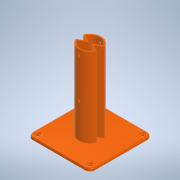
# Autodesk Inventor part: Arduino_case_top_JC_Rev1
Saved by Autodesk Inventor 2020 (Build 240168000, 168)
## iProperties
Created: 2019-08-28
Part Number: Arduino_case_top_JC_Rev1
Material: Generic
Document SubType Name: Modeling
Designer: jcocker
Density: 1 g/cm^3
Appearance: Smooth - Light Orange
Author: jcocker
Autodesk Inventor part; units mm, degrees
ref_plane "YZ Plane" through (0, 0, 0) normal (1, 0, 0) x (0, 1, 0)
ref_plane "XZ Plane" through (0, 0, 0) normal (0, 1, 0) x (-1, 0, 0)
ref_plane "XY Plane" through (0, 0, 0) normal (0, 0, 1) x (1, 0, 0)
sketch "Sketch1" plane through (0, 0, 0) normal (0, 1, 0) x (-1, 0, 0)
  circle A0 centre (0, 0) radius 14.2875
  line L0 (5.08, 0) -> (13.4462, -4.8303)
  line L1 (5.08, 0) -> (14.7405, 0) construction
  line L2 (5.08, 0) -> (13.4462, 4.8303)
  line L3 (-5.08, 0) -> (-13.4462, -4.8303)
  line L4 (-5.08, 0) -> (-13.4462, 4.8303)
  dimension "d0" = 28.575
  dimension "d1" = 5.08
  dimension "d2" = 30
  constraints: 10 end point, 1 coincident, 1 equal length, 1 horizontal, 1 symmetric about line, 3 other
  measures "d1" distance of point (0, 0) L0.start
  measures "d2" angle of L0 L1
extrude "Extrusion1" add sketch "Sketch1" along normal blind 101.6 contours L2 L0 A0 L3 L4
shell "Shell1" thickness 1.7 removed faces 2 at (0, 0, -4.7625) at (0, 101.6, -4.7625)
sketch "Sketch2" plane through (0, 0, 0) normal (0, -1, 0) x (1, 0, 0)
  line L0 (33.65, 40) -> (-33.65, 40)
  line L1 (-40, 33.65) -> (-40, -33.65)
  line L2 (-33.65, -40) -> (33.65, -40)
  line L3 (40, -33.65) -> (40, 33.65)
  line L4 (40, 40) -> (-40, -40) construction
  line L5 (-40, 40) -> (40, -40) construction
  arc A0 (33.65, -40) -> (40, -33.65) centre (33.65, -33.65) ccw
  arc A1 (40, 33.65) -> (33.65, 40) centre (33.65, 33.65) ccw
  arc A2 (-33.65, 40) -> (-40, 33.65) centre (-33.65, 33.65) ccw
  arc A3 (-40, -33.65) -> (-33.65, -40) centre (-33.65, -33.65) ccw
  point P0 (0, 0)
  dimension "d6" = 80
  dimension "d7" = 80
  dimension "d9" = 6.35
  constraints: 12 end point, 8 point on circle, 8 point on line, 8 tangent, 4 centre point, 3 equal radius, 2 midpoint, 2 parallel, 1 horizontal, 1 perpendicular
  measures "d6" distance of L5.end L4.end
  measures "d7" distance of L4.end L5.start
  measures "d9" radius of A0
extrude "Extrusion2" add sketch "Sketch2" along normal blind 3.175
sketch "Sketch3" plane through (0, 0, 0) normal (0, 1, 0) x (1, 0, 0)
  arc A0 (-11.2968, -5.5523) -> (11.2968, -5.5523) centre (0, 0) ccw projected
  line L0 (11.2968, -5.5523) -> (1.68, 0) projected
  line L1 (1.68, 0) -> (11.2968, 5.5523) projected
  arc A1 (11.2968, 5.5523) -> (-11.2968, 5.5523) centre (0, 0) ccw projected
  line L2 (-11.2968, 5.5523) -> (-1.68, 0) projected
  line L3 (-1.68, 0) -> (-11.2968, -5.5523) projected
extrude "Extrusion3" cut sketch "Sketch3" against normal through all
sketch "Sketch4" plane through (0, 0, 0) normal (0, 0, 1) x (1, 0, 0)
  circle A0 centre (0, 44.45) radius 1.5875
  point P0 (0, 0)
  dimension "d14" = 3.175
  dimension "d15" = 44.45
  constraints: 1 centre point
  measures "d14" diameter of A0
  measures "d15" distance of point (0, 0) A0.centre
extrude "Extrusion4" cut sketch "Sketch4" along normal mid plane 101.6
sketch "Sketch5" plane through (0, 0, 0) normal (0, 0, 1) x (1, 0, 0)
  circle A0 centre (0, 95.25) radius 1.5875
  line L0 (33.65, 0) -> (40, 0) projected
  point P0 (0, 0)
  dimension "d18" = 3.175
  dimension "d19" = 95.25
  constraints: 1 centre point
  measures "d18" diameter of A0
  measures "d19" distance from line of L0 A0.centre
extrude "Extrusion5" cut sketch "Sketch5" along normal blind 101.6 and the other way blind 50.8
sketch "Sketch6" plane through (0, 0, 0) normal (0, 1, 0) x (1, 0, 0)
  arc A0 (40, 33.65) -> (33.65, 40) centre (33.65, 33.65) ccw projected
  circle A1 centre (33.65, 33.65) radius 1.7
  point P0 (0, 0)
  dimension "d24" = 3.4
  constraints: 1 centre point, 1 coincident
  measures "d24" diameter of A1
extrude "Extrusion6" cut sketch "Sketch6" against normal blind 25.4
sketch "Sketch7" plane through (0, 0, 0) normal (0, 1, 0) x (1, 0, 0)
  arc A0 (40, 33.65) -> (33.65, 40) centre (33.65, 33.65) ccw projected
  circle A1 centre (33.65, 33.65) radius 3.175
  point P0 (0, 0)
  dimension "d27" = 6.35
  constraints: 1 centre point, 1 coincident
  measures "d27" diameter of A1
extrude "Extrusion7" cut sketch "Sketch7" against normal blind 1.27
mirror "Mirror1" about plane through (0, 0, 0) normal (1, 0, 0) of "Extrusion6", "Extrusion7"
mirror "Mirror2" about plane through (0, 0, 0) normal (0, 0, 1) of "Extrusion6", "Extrusion7", "Mirror1"
fillet "Fillet1" radius 1.5875 8 edges at (-38.1401, 0, -38.1401) (0, 0, -40) (38.1401, 0, -38.1401) (40, 0, 0) (38.1401, 0, 38.1401) (0, 0, 40) (-38.1401, 0, 38.1401) (-40, 0, 0)
fillet "Fillet2" radius 0.635 8 edges at (-30.475, 0, 33.65) (-30.475, 0, -33.65) (30.475, 0, -33.65) (30.475, 0, 33.65) (-13.4462, 50.8, 4.8303) (-13.4462, 50.8, -4.8303) (13.4462, 50.8, 4.8303) (13.4462, 50.8, -4.8303)
body "Solid1"
